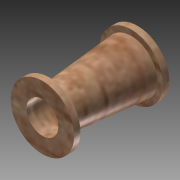
# Autodesk Inventor part: 带轮
Saved by Autodesk Inventor 2013 (Build 170138000, 138)
## iProperties
Created: 2012-10-03
Part Number: 带轮
Material: 木材(桦木)
Document SubType Name: Modeling
Designer: Zhensheng
Density: 0.55 g/cm^3
Mass: 30.1708 g
Surface Area: 93.0227 cm^2
Volume: 54.856 cm^3
Author: Zhensheng
Autodesk Inventor part; units mm, degrees
ref_plane "YZ Plane" through (0, 0, 0) normal (1, 0, 0) x (0, 1, 0)
ref_plane "XZ Plane" through (0, 0, 0) normal (0, 1, 0) x (-1, 0, 0)
ref_plane "XY Plane" through (0, 0, 0) normal (0, 0, 1) x (1, 0, 0)
sketch "草图1" plane through (0, 0, 0) normal (0, 1, 0) x (-1, 0, 0)
  circle A0 centre (0, 0) radius 6
  dimension "带轮直径" = 12
  constraints: 1 centre point, 1 coincident
  measures "带轮直径" diameter of A0
extrude "拉伸2" add sketch "草图1" along normal blind 26 draft 5
sketch "草图3" plane through (0, 0, 0) normal (0, -1, 0) x (1, 0, 0)
  circle A0 centre (0, 0) radius 10
  dimension "外径" = 20
  constraints: 1 centre point, 1 coincident
  measures "外径" diameter of A0
sketch "草图4" plane through (0, 26, 0) normal (0, 1, 0) x (1, 0, 0)
  circle A0 centre (0, 0) radius 10
  dimension "d12" = 20
  constraints: 1 centre point, 1 coincident
  measures "d12" diameter of A0
extrude "拉伸4" add sketch "草图3" along normal blind 2
extrude "拉伸5" add sketch "草图4" along normal blind 2
sketch "草图2" plane through (0, 0, 0) normal (0, -1, 0) x (1, 0, 0)
  circle A0 centre (0, 0) radius 5
  dimension "孔径" = 10
  constraints: 1 centre point, 1 coincident
  measures "孔径" diameter of A0
extrude "拉伸3" cut sketch "草图2" along normal through all both and the other way through all
equation "\"d12\" = 外径"
equation "\"d15\" = 外圆"
equation "\"外圆\" = 2"
